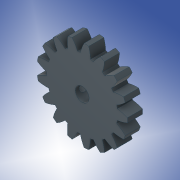
# Autodesk Inventor part: Motor Gear
Saved by Autodesk Inventor 2017 SP1 (Build 210196100, 196)
## iProperties
Created: 2017-07-05
Part Number: Motor Gear
Material: ABS Plastic
Document SubType Name: Modeling
Designer: zallen
Density: 1.06 g/cm^3
Appearance: CR Dark Blue
Author: zallen
Autodesk Inventor part; units mm, degrees
ref_plane "YZ Plane" through (0, 0, 0) normal (1, 0, 0) x (0, 1, 0)
ref_plane "XZ Plane" through (0, 0, 0) normal (0, 1, 0) x (-1, 0, 0)
ref_plane "XY Plane" through (0, 0, 0) normal (0, 0, 1) x (1, 0, 0)
sketch "Sketch1" plane through (0, 0, 0) normal (0, 0, 1) x (1, 0, 0)
  circle A0 centre (0, 0) radius 14
  line L0 (0, 0) -> (16, 0) construction
  arc A1 (17.8564, 0.9) -> (13.8564, 2) centre (11.9173, -12.8741) ccw
  arc A2 (13.8564, -2) -> (17.8564, -0.9) centre (11.9173, 12.8741) ccw
  arc A3 (13.8564, -2) -> (13.8564, 2) centre (0, 0) ccw
  arc A4 (17.8564, -0.9) -> (17.8564, 0.9) centre (-2.1233, 0) ccw
  arc A5 (16.3255, 7.2897) -> (12.1982, 6.8705) centre (15.7632, -7.6998) ccw
  arc A6 (16.9757, 5.6113) -> (16.3255, 7.2897) centre (-1.9799, -0.767) ccw
  arc A7 (13.6432, 3.1406) -> (16.9757, 5.6113) centre (6.4619, 16.3098) ccw
  arc A8 (13.6432, 3.1406) -> (12.1982, 6.8705) centre (0, 0) ccw
  arc A9 (12.5897, 12.6949) -> (8.8926, 10.813) centre (17.4802, -1.4855) ccw
  arc A10 (13.8024, 11.3647) -> (12.5897, 12.6949) centre (-1.5692, -1.4305) ccw
  arc A11 (11.5874, 7.857) -> (13.8024, 11.3647) centre (0.1337, 17.5427) ccw
  arc A12 (11.5874, 7.857) -> (8.8926, 10.813) centre (0, 0) ccw
  arc A13 (7.1536, 16.3856) -> (4.386, 13.2952) centre (16.8364, 4.9294) ccw
  arc A14 (8.7649, 15.5832) -> (7.1536, 16.3856) centre (-0.9465, -1.9007) ccw
  arc A15 (7.9667, 11.5123) -> (8.7649, 15.5832) centre (-6.2125, 16.4064) ccw
  arc A16 (7.9667, 11.5123) -> (4.386, 13.2952) centre (0, 0) ccw
  arc A17 (0.7514, 17.8633) -> (-0.713, 13.9818) centre (13.9188, 10.6786) ccw
  arc A18 (2.5437, 17.6972) -> (0.7514, 17.8633) centre (-0.1959, -2.1143) ccw
  arc A19 (3.27, 13.6128) -> (2.5437, 17.6972) centre (-11.7196, 13.0543) ccw
  arc A20 (3.27, 13.6128) -> (-0.713, 13.9818) centre (0, 0) ccw
  arc A21 (-5.7523, 16.9285) -> (-5.7156, 12.7801) centre (9.1214, 14.9855) ccw
  arc A22 (-4.021, 17.421) -> (-5.7523, 16.9285) centre (0.5811, -2.0423) ccw
  arc A23 (-1.8683, 13.8748) -> (-4.021, 17.421) centre (-15.644, 7.9392) ccw
  arc A24 (-1.8683, 13.8748) -> (-5.7156, 12.7801) centre (0, 0) ccw
  arc A25 (-11.4791, 13.7073) -> (-9.9464, 9.8524) centre (3.092, 17.2686) ccw
  arc A26 (-10.0427, 14.7921) -> (-11.4791, 13.7073) centre (1.2796, -1.6945) ccw
  arc A27 (-6.7543, 12.2629) -> (-10.0427, 14.7921) centre (-17.4555, 1.7518) ccw
  arc A28 (-6.7543, 12.2629) -> (-9.9464, 9.8524) centre (0, 0) ccw
  arc A29 (-15.6556, 8.635) -> (-12.8338, 5.594) centre (-3.3549, 17.2194) ccw
  arc A30 (-14.708, 10.1654) -> (-15.6556, 8.635) centre (1.8053, -1.1178) ccw
  arc A31 (-10.7281, 8.9949) -> (-14.708, 10.1654) centre (-16.9096, -4.6722) ccw
  arc A32 (-10.7281, 8.9949) -> (-12.8338, 5.594) centre (0, 0) ccw
  arc A33 (-17.7177, 2.3964) -> (-13.988, 0.5802) centre (-9.3487, 14.8447) ccw
  arc A34 (-17.387, 4.1658) -> (-17.7177, 2.3964) centre (2.0872, -0.3902) ccw
  arc A35 (-13.253, 4.5121) -> (-17.387, 4.1658) centre (-14.08, -10.4651) ccw
  arc A36 (-13.253, 4.5121) -> (-13.988, 0.5802) centre (0, 0) ccw
  arc A37 (-17.387, -4.1658) -> (-13.253, -4.5121) centre (-14.08, 10.4651) ccw
  arc A38 (-17.7177, -2.3964) -> (-17.387, -4.1658) centre (2.0872, 0.3902) ccw
  arc A39 (-13.988, -0.5802) -> (-17.7177, -2.3964) centre (-9.3487, -14.8447) ccw
  arc A40 (-13.988, -0.5802) -> (-13.253, -4.5121) centre (0, 0) ccw
  arc A41 (-14.708, -10.1654) -> (-10.7281, -8.9949) centre (-16.9096, 4.6722) ccw
  arc A42 (-15.6556, -8.635) -> (-14.708, -10.1654) centre (1.8053, 1.1178) ccw
  arc A43 (-12.8338, -5.594) -> (-15.6556, -8.635) centre (-3.3549, -17.2194) ccw
  arc A44 (-12.8338, -5.594) -> (-10.7281, -8.9949) centre (0, 0) ccw
  arc A45 (-10.0427, -14.7921) -> (-6.7543, -12.2629) centre (-17.4555, -1.7518) ccw
  arc A46 (-11.4791, -13.7073) -> (-10.0427, -14.7921) centre (1.2796, 1.6945) ccw
  arc A47 (-9.9464, -9.8524) -> (-11.4791, -13.7073) centre (3.092, -17.2686) ccw
  arc A48 (-9.9464, -9.8524) -> (-6.7543, -12.2629) centre (0, 0) ccw
  arc A49 (-4.021, -17.421) -> (-1.8683, -13.8748) centre (-15.644, -7.9392) ccw
  arc A50 (-5.7523, -16.9285) -> (-4.021, -17.421) centre (0.5811, 2.0423) ccw
  arc A51 (-5.7156, -12.7801) -> (-5.7523, -16.9285) centre (9.1214, -14.9855) ccw
  arc A52 (-5.7156, -12.7801) -> (-1.8683, -13.8748) centre (0, 0) ccw
  arc A53 (2.5437, -17.6972) -> (3.27, -13.6128) centre (-11.7196, -13.0543) ccw
  arc A54 (0.7514, -17.8633) -> (2.5437, -17.6972) centre (-0.1959, 2.1143) ccw
  arc A55 (-0.713, -13.9818) -> (0.7514, -17.8633) centre (13.9188, -10.6786) ccw
  arc A56 (-0.713, -13.9818) -> (3.27, -13.6128) centre (0, 0) ccw
  arc A57 (8.7649, -15.5832) -> (7.9667, -11.5123) centre (-6.2125, -16.4064) ccw
  arc A58 (7.1536, -16.3856) -> (8.7649, -15.5832) centre (-0.9465, 1.9007) ccw
  arc A59 (4.386, -13.2952) -> (7.1536, -16.3856) centre (16.8364, -4.9294) ccw
  arc A60 (4.386, -13.2952) -> (7.9667, -11.5123) centre (0, 0) ccw
  arc A61 (13.8024, -11.3647) -> (11.5874, -7.857) centre (0.1337, -17.5427) ccw
  arc A62 (12.5897, -12.6949) -> (13.8024, -11.3647) centre (-1.5692, 1.4305) ccw
  arc A63 (8.8926, -10.813) -> (12.5897, -12.6949) centre (17.4802, 1.4855) ccw
  arc A64 (8.8926, -10.813) -> (11.5874, -7.857) centre (0, 0) ccw
  arc A65 (16.9757, -5.6113) -> (13.6432, -3.1406) centre (6.4619, -16.3098) ccw
  arc A66 (16.3255, -7.2897) -> (16.9757, -5.6113) centre (-1.9799, 0.767) ccw
  arc A67 (12.1982, -6.8705) -> (16.3255, -7.2897) centre (15.7632, 7.6998) ccw
  arc A68 (12.1982, -6.8705) -> (13.6432, -3.1406) centre (0, 0) ccw
  point P0 (17.8767, 0)
  point P1 (16.6695, 6.4578)
  point P2 (13.211, 12.0434)
  point P3 (7.9683, 16.0025)
  point P4 (1.6495, 17.8004)
  point P5 (-4.8922, 17.1942)
  point P6 (-10.7731, 14.2659)
  point P7 (-15.199, 9.4109)
  point P8 (-17.5723, 3.2848)
  point P9 (-17.5723, -3.2848)
  point P10 (-15.199, -9.4109)
  point P11 (-10.7731, -14.2659)
  point P12 (-4.8922, -17.1942)
  point P13 (1.6495, -17.8004)
  point P14 (7.9683, -16.0025)
  point P15 (13.211, -12.0434)
  point P16 (16.6695, -6.4578)
  dimension "d0" = 28
  dimension "d1" = 16
  dimension "d2" = 15
  dimension "d3" = 4
  dimension "d4" = 2
  dimension "d6" = 1.8
  dimension "d15" = 20
  dimension "d18" = 360
  constraints: 137 point on circle, 68 centre point, 3 symmetric about line, 2 end point, 1 coincident, 1 horizontal, 1 point on line, 228 other
  measures "d1" distance of L0.start L0.end
  measures "d2" radius of A1
  measures "d3" horizontal distance of A1.start A1.end
  measures "d4" distance from line of L0 A1.end
  measures "d6" distance of A2.end A1.start
  measures "d15" radius of A4
extrude "Extrusion1" add sketch "Sketch1" along normal blind 6
sketch "Sketch5" plane through (0, 0, 6) normal (0, 0, 1) x (1, 0, 0)
  circle A0 centre (0, 0) radius 2.75
  dimension "d32" = 5.5
  constraints: 1 centre point, 1 coincident
  measures "d32" diameter of A0
extrude "Extrusion5" cut sketch "Sketch5" against normal through all
sketch "Sketch8" plane through (0, 0, 0) normal (1, 0, 0) x (0, 1, 0)
  circle A0 centre (-0.25, 3) radius 1.5
  line L0 (-2.75, 6) -> (-2.75, 0) projected
  point P0 (0, 0)
  point P1 (-2.75, 3)
  dimension "d38" = 3
  dimension "d39" = 0.25
  constraints: 1 centre point, 1 horizontal alignment, 1 midpoint
  measures "d38" diameter of A0
  measures "d39" horizontal distance of point (0, 0) A0.centre
extrude "Extrusion7" cut sketch "Sketch8" against normal through all
body "Solid1"
